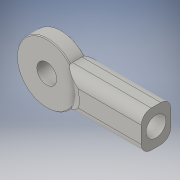
# Autodesk Inventor part: .125 in female rod end
Saved by Autodesk Inventor 2016 (Build 200138000, 138)
## iProperties
Created: 2015-10-31
Part Number: .125 in female rod end
Material: Generic
Document SubType Name: Modeling
Designer: Delta
Density: 1 g/cm^3
Appearance: Default
Author: Delta
Autodesk Inventor part; units mm, degrees
ref_plane "YZ Plane" through (0, 0, 0) normal (1, 0, 0) x (0, 1, 0)
ref_plane "XZ Plane" through (0, 0, 0) normal (0, 1, 0) x (-1, 0, 0)
ref_plane "XY Plane" through (0, 0, 0) normal (0, 0, 1) x (1, 0, 0)
sketch "Sketch1" plane through (0, 0, 0) normal (0, 0, 1) x (1, 0, 0)
  line L0 (3.0039, 0) -> (42.926, 0)
  line L1 (42.926, 0) -> (42.926, 11.684)
  line L2 (42.926, 11.684) -> (8.3054, 11.684)
  line L3 (3.0039, 8.6681) -> (3.0039, 0)
  line L4 (3.0039, 8.6681) -> (8.3054, 11.684)
  dimension "d1" = 11.684
  constraints: 10 end point, 2 perpendicular, 1 horizontal, 1 parallel
  measures "d1" distance of L1.end L0.end
extrude "Extrusion3" add sketch "Sketch1" along normal blind 9.398
sketch "Sketch3" plane through (0, 0, 9.398) normal (0, 0, 1) x (1, 0, 0)
  circle A0 centre (10.3855, 5.3641) radius 9.652
  line L0 (42.926, 0) -> (42.926, 11.684) projected
  line L1 (42.926, 5.3641) -> (20.066, 5.3641)
  line L2 (42.926, 5.3641) -> (65.786, 5.3641) construction
  point P0 (0, 0)
  dimension "d11" = 19.304
  dimension "d12" = 22.86
  dimension "d13" = 180
  constraints: 4 end point, 1 centre point, 1 collinear, 1 horizontal, 1 perpendicular, 1 point on line
  measures "d11" diameter of A0
  measures "d12" distance of L1.start L1.end
  measures "d13" angle of L1 L2
extrude "Extrusion4" add sketch "Sketch3" against normal blind 9.398
sketch "Sketch5" plane through (0, 0, 9.398) normal (0, 0, 1) x (1, 0, 0)
  line L0 (42.926, 11.684) -> (17.6806, 11.684) projected
  line L1 (17.6806, 11.684) -> (17.6806, 11.684)
  line L2 (17.6806, 11.684) -> (17.6806, 11.684) construction
  circle A0 centre (10.3618, 5.3594) radius 9.6737
  line L3 (17.6806, 11.684) -> (17.6806, 11.684)
  point P0 (0, 0)
  dimension "d18" = 90
  constraints: 6 end point, 1 centre point, 1 horizontal, 1 perpendicular, 1 vertical
  measures "d18" angle of L1 L2
extrude "Extrusion6" cut sketch "Sketch5" against normal blind 2.3368
sketch "Sketch6" plane through (0, 0, 0) normal (0, 0, -1) x (-1, 0, 0)
  arc A0 (-18.4097, 0) -> (-17.6806, 11.684) centre (-10.3855, 5.3641) ccw projected
  line L0 (-10.3855, 15.0161) -> (-10.3855, -4.2879)
  circle A1 centre (-10.3855, 5.3641) radius 9.652
  point P0 (0, 0)
  constraints: 2 end point, 2 point on circle, 1 centre point, 1 coincident, 1 concentric, 1 vertical
extrude "Extrusion7" cut sketch "Sketch6" against normal blind 2.3368
sketch "Sketch7" plane through (42.926, 0, 0) normal (1, 0, 0) x (0, 0, -1)
  line L0 (0, 11.684) -> (-9.398, 11.684) projected
  line L1 (0, 11.684) -> (-9.398, 11.684)
  line L2 (-4.699, 11.684) -> (-4.699, 0)
  line L3 (0, 0) -> (-9.398, 0) projected
  circle A0 centre (-4.699, 5.842) radius 3.175
  dimension "d23" = 6.35
  constraints: 4 end point, 3 midpoint, 1 centre point, 1 collinear
  measures "d23" diameter of A0
extrude "Extrusion8" cut sketch "Sketch7" against normal blind 17.78
sketch "Sketch8" plane through (0, 0, 2.3368) normal (0, 0, -1) x (-1, 0, 0)
  arc A0 (-18.4097, 0) -> (-17.6806, 11.684) centre (-10.3855, 5.3641) ccw projected
  line L0 (-10.3855, -4.2879) -> (-10.3855, 15.0161)
  circle A1 centre (-10.3855, 5.3641) radius 3.175
  point P0 (0, 0)
  point P1 (-17.7767, 11.5714)
  point P2 (-18.4839, 0.1126)
  dimension "d27" = 6.35
  constraints: 2 end point, 2 point on circle, 1 centre point, 1 coincident, 1 vertical
  measures "d27" diameter of A1
extrude "Extrusion9" cut sketch "Sketch8" against normal blind 17.78 contours A1 L0 | L0 A1
fillet "Fillet4" radius 3.175 6 edges at (30.6678, 0, 0) (30.6706, 0, 9.398) (20.0187, 5.9651, 0) (30.3033, 11.684, 0) (20.0164, 5.9656, 9.398) (30.3038, 11.684, 9.398)
fillet "Fillet5" radius 0.254 2 edges at (0.7518, 4.7696, 2.3368) (0.7518, 4.7696, 7.0612)
body "Solid1"
